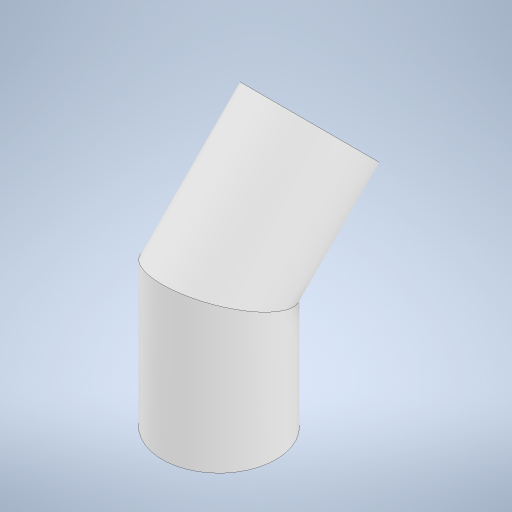
# Autodesk Inventor part: Semicodo
Saved by Autodesk Inventor 2024 (Build 280153000, 153)
## iProperties
Created: 2023-02-27
Part Number: Semicodo
Material: Genérico
Document SubType Name: Modeling
Designer: Braya
Density: 1 g/cm^3
Appearance: Suave - Blanco
Mass: 18.385 g
Surface Area: 121.761 cm^2
Volume: 18.385 cm^3
Author: Braya
Autodesk Inventor part; units mm, degrees
ref_plane "YZ Plane" through (0, 0, 0) normal (1, 0, 0) x (0, 1, 0)
ref_plane "XZ Plane" through (0, 0, 0) normal (0, 1, 0) x (-1, 0, 0)
sketch "Boceto1" plane through (0, 0, 0) normal (1, 0, 0) x (0, 1, 0)
  line L0 (0, 0) -> (30, 0)
  line L1 (0, 0) -> (30, 0) construction
  line L2 (30, 0) -> (51.2132, -21.2132)
  line L3 (0, 0) -> (0, -12)
  line L4 (0, -12) -> (25.0294, -12)
  line L5 (51.2132, -21.2132) -> (42.7279, -29.6985)
  line L6 (42.7279, -29.6985) -> (25.0294, -12)
  line L7 (0, 0) -> (0, -13.325)
  line L8 (51.2132, -21.2132) -> (41.791, -30.6354)
  line L9 (41.791, -30.6354) -> (24.4806, -13.325)
  line L10 (0, -13.325) -> (24.4806, -13.325)
  line L11 (24.4806, -13.325) -> (24.4806, -12)
  line L12 (24.4806, -13.325) -> (25.4175, -12.3881)
  line L13 (0, 0) -> (30, 0)
  line L14 (51.2132, -21.2132) -> (30, 0)
  point P0 (0, -12)
  dimension "d0" = 30
  dimension "d1" = 0
  dimension "d2" = 30
  dimension "d3" = 135
  dimension "d4" = 12
  dimension "d5" = 12
  dimension "d6" = 13.325
  dimension "d7" = 13.325
  constraints: 30 end point, 7 perpendicular, 4 point on line, 3 collinear, 2 horizontal
  measures "d0" distance of L0.start L0.end
  measures "d1" distance between parallel lines of L0 L1
  measures "d2" distance of L0.end L2.end
  measures "d3" angle of L0 L2
  measures "d4" distance of L0.start L3.end
  measures "d5" distance of L2.end L5.end
  measures "d6" distance of L0.start L7.end
  measures "d7" distance of L2.end L8.end
revolve "Revolución1" add sketch "Boceto1" angle 360 about axis through (0, 0, 0) along (0, 1, 0) contours L4 L11 L10 L7
revolve "Revolución2" add sketch "Boceto1" angle 360 about axis through (0, 30, 0) along (0, 0.7071, -0.7071) contours L8 L9 L12 L6
ref_plane "Plano de trabajo1" through (0, 24.4806, -13.325) normal (0, 0.9239, -0.3827) x (-1, 0, 0)
sketch "Boceto6" plane through (0, 24.4806, 0) normal (0, 1, 0) x (1, 0, 0)
  circle A0 centre (0, 0) radius 13.325 projected
  circle A1 centre (0, 0) radius 12 projected
  point P0 (0, 13.325)
  constraints: 1 vertical alignment
sketch "Boceto7" plane through (0, 33.9028, -3.9028) normal (0, -0.7071, 0.7071) x (1, 0, 0)
  circle A0 centre (0, 0) radius 13.325 projected
  circle A1 centre (0, 0) radius 12 projected
  point P0 (0, -21.2132)
  point P1 (0, -13.325)
  constraints: 1 vertical alignment
extrude "Extrusión3" add sketch "Boceto6" along normal up to surface surface through (0, 24.4806, -13.325) normal (0, 0.9239, -0.3827)
extrude "Extrusión4" add sketch "Boceto7" along normal up to surface surface through (0, 24.4806, -13.325) normal (0, 0.9239, -0.3827)
fillet "Empalme1" [suppressed]
